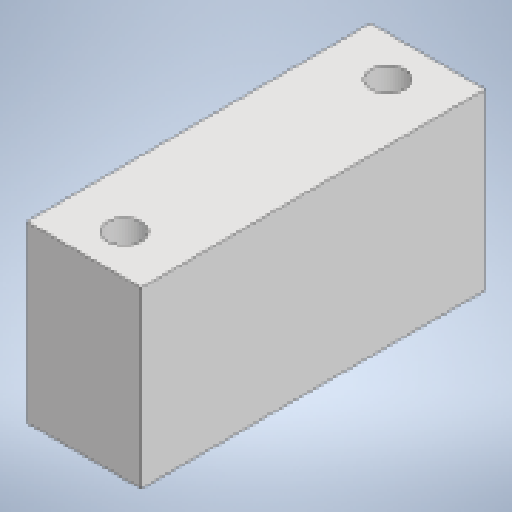
# Autodesk Inventor part: BF12_Spacer
Saved by Autodesk Inventor 2023 (Build 270158000, 158)
## iProperties
Created: 2022-05-01
Part Number: BF12_Spacer
Material: Generic
Document SubType Name: Modeling
Designer: plebbb
Density: 1 g/cm^3
Appearance: Default
Author: plebbb
Autodesk Inventor part; units mm, degrees
ref_plane "YZ Plane" through (0, 0, 0) normal (1, 0, 0) x (0, 1, 0)
ref_plane "XZ Plane" through (0, 0, 0) normal (0, 1, 0) x (-1, 0, 0)
ref_plane "XY Plane" through (0, 0, 0) normal (0, 0, 1) x (1, 0, 0)
sketch "Sketch1" plane through (0, 0, 0) normal (0, 1, 0) x (-1, 0, 0)
  line L0 (0, 0) -> (20, 0)
  line L1 (20, 0) -> (20, -60)
  line L2 (20, -60) -> (0, -60)
  line L3 (0, -60) -> (0, 0)
  circle A0 centre (10, -53) radius 3
  circle A1 centre (10, -7) radius 3
  line L4 (10, -7) -> (10, -53) construction
  point P0 (10, 0)
  point P1 (10, -60)
  point P2 (20, -30)
  point P3 (10, -30)
  dimension "d0" = 60
  dimension "d1" = 20
  dimension "d2" = 6
  dimension "d3" = 6
  dimension "d4" = 46
  constraints: 10 end point, 4 midpoint, 2 centre point, 2 parallel, 2 vertical alignment, 1 coincident, 1 horizontal, 1 horizontal alignment, 1 perpendicular, 1 vertical
  measures "d0" distance of L0.end L1.end
  measures "d1" distance of L1.end L2.end
  measures "d2" diameter of A1
  measures "d3" diameter of A0
  measures "d4" distance of L4.start L4.end
extrude "Extrusion1" add sketch "Sketch1" along normal blind 30.4
sketch "Sketch2" plane through (-20, 0, 0) normal (0, 0, 1) x (1, 0, 0)
  line L0 (0, 0) -> (20, 0) projected
  line L1 (20, 0) -> (20, 30.4) projected
  line L2 (0, 30.4) -> (20, 30.4) projected
  line L3 (0, 0) -> (0, 30.4) projected
extrude "Extrusion2" add sketch "Sketch2" along normal blind 2.917
body "Solid1"
